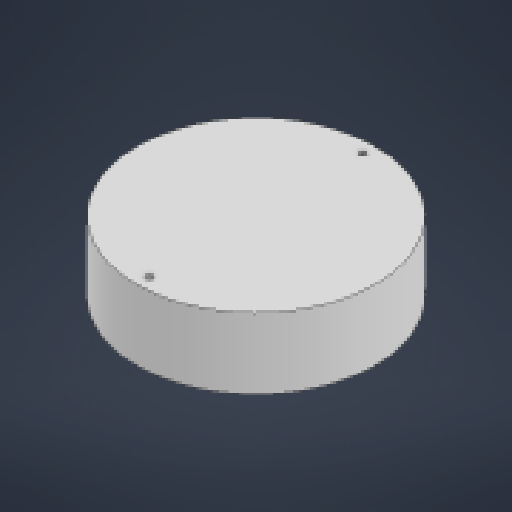
# Autodesk Inventor part: Capsule
Saved by Autodesk Inventor 2025 (Build 290162000, 162)
## iProperties
Created: 2024-07-01
Part Number: Capsule
Material: Generic
Document SubType Name: Modeling
Designer: mayhe
Density: 1 g/cm^3
Appearance: Default
Author: mayhe
Autodesk Inventor part; units mm, degrees
ref_plane "YZ Plane" through (0, 0, 0) normal (1, 0, 0) x (0, 1, 0)
ref_plane "XZ Plane" through (0, 0, 0) normal (0, 1, 0) x (-1, 0, 0)
ref_plane "XY Plane" through (0, 0, 0) normal (0, 0, 1) x (1, 0, 0)
sketch "Sketch1" plane through (0, 0, 0) normal (0, 1, 0) x (-1, 0, 0)
  circle A0 centre (0, 0) radius 85
  circle A1 centre (0, 0) radius 80
  dimension "d0" = 170
  dimension "d1" = 160
  constraints: 2 centre point, 2 coincident
  measures "d0" diameter of A0
  measures "d1" diameter of A1
extrude "Extrusion1" add sketch "Sketch1" along normal blind 10 contours A0 | A1
extrude "Extrusion2" add sketch "Sketch1" along normal blind 50
sketch "Sketch2" plane through (0, 50, 0) normal (0, 1, 0) x (1, 0, 0)
  circle A0 centre (0, 0) radius 85
  constraints: 1 centre point, 1 coincident
extrude "Extrusion3" add sketch "Sketch2" against normal blind 10
sketch "Sketch3" plane through (0, 50, 0) normal (0, 1, 0) x (1, 0, 0)
  circle A0 centre (0, 0) radius 76
  circle A1 centre (0, -76) radius 2.25
  circle A2 centre (0, 76) radius 2.25
  dimension "d8" = 152
  dimension "d9" = 4.5
  dimension "d10" = 4.5
  constraints: 3 centre point, 2 point on circle, 1 coincident
  measures "d8" diameter of A0
  measures "d9" diameter of A1
  measures "d10" diameter of A2
extrude "Extrusion4" cut sketch "Sketch3" against normal blind 10 contours A2 A0 | A0 A2 | A1 A0 | A0 A1
sketch "Sketch4" plane through (0, 0, 0) normal (0, -1, 0) x (1, 0, 0)
  circle A0 centre (0, -76) radius 2.25 projected
  circle A1 centre (0, 0) radius 76
  circle A2 centre (0, 76) radius 2.25
  constraints: 2 centre point, 2 point on circle, 1 coincident
extrude "Extrusion5" cut sketch "Sketch4" against normal blind 10 contours A2 A1 | A1 A2
body "Solid1"
